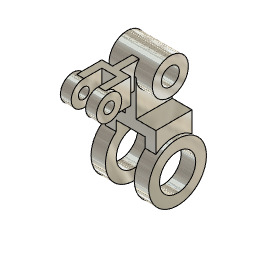
Exercise-5 v0 (Autodesk Fusion 360 design; units mm, degrees)
Autodesk Fusion 360 part; units mm, degrees
sketch "Sketch1" plane through (0, 0, 0) normal (1, 0, 0) x (0, 1, 0)
  circle A0 centre (0, 0) radius 25
  circle A1 centre (0, 0) radius 40
  circle A2 centre (0, 110) radius 12.5
  circle A3 centre (0, 110) radius 25
  circle A4 centre (-80, 110) radius 7.5
  circle A5 centre (-80, 110) radius 17.5
  dimension "d1" = 50
  dimension "d2" = 80
  dimension "d3" = 25
  dimension "d4" = 50
  dimension "d5" = 110
  dimension "d6" = 15
  dimension "d7" = 35
  dimension "d8" = 80
  constraint coincident A0.centre A1.centre
  constraint concentric A2 A3
  constraint concentric A4 A5
  measures "d1" diameter of A0
  measures "d2" diameter of A1
  measures "d3" diameter of A2
  measures "d4" diameter of A3
  measures "d5" distance of A0.centre A2.centre
  measures "d6" diameter of A4
  measures "d7" diameter of A5
  measures "d8" distance of A2.centre A4.centre
extrude "Extrude1" add sketch "Sketch1" along normal blind 20 from surface at 20 contours A1 makes body 1
extrude "Extrude2" add sketch "Sketch1" along normal blind 15 from surface at 10 separate body contours A5 makes body 2
extrude "Extrude3" add sketch "Sketch1" along normal mid plane 60 separate body contours A3 makes body 3
mirror "Mirror1" about plane through (0, 0, 0) normal (1, 0, 0) of bodies 2 1 makes body 4 at (-33.3333, 39.9503, -1.9938) makes body 5 at (-20, -62.587, 108.2576)
sketch "Sketch2" plane through (0, 0, 0) normal (0, 1, 0) x (1, 0, 0)
  line L0 (-40, -40) -> (-40, 40)
  line L1 (-20, -40) -> (-20, 40)
  line L2 (40, -40) -> (40, 40)
  line L3 (20, -40) -> (20, 40)
  line L4 (-30, -85) -> (-30, -135)
  line L5 (30, -135) -> (30, -85)
  line L6 (-20, 0) -> (-35, 0)
  line L7 (-35, 0) -> (-35, -45)
  line L8 (-35, -45) -> (-20, -45)
  line L9 (-20, -45) -> (-20, 0)
  line L10 (0, 0) -> (0, -67.4889) construction
  line L11 (35, -45) -> (20, -45)
  line L12 (35, 0) -> (35, -45)
  line L13 (20, -45) -> (20, 0)
  line L14 (20, 0) -> (35, 0)
  line L15 (-35, -45) -> (35, -45)
  line L16 (35, -45) -> (35, -60)
  line L17 (35, -60) -> (-35, -60)
  line L18 (-35, -60) -> (-35, -45)
  line L19 (-7.5, -45) -> (7.5, -45)
  line L20 (7.5, -45) -> (7.5, -110)
  line L21 (7.5, -110) -> (-7.5, -110)
  line L22 (-7.5, -110) -> (-7.5, -45)
  dimension "d19" = 15
  dimension "d20" = 45
  dimension "d21" = 15
  dimension "d22" = 15
  dimension "d23" = 65
  dimension "d24" = 27.5
  constraint horizontal L6
  constraint vertical L7
  constraint horizontal L8
  constraint vertical L9
  constraint midpoint L1 L6.start
  constraint coincident L10.start origin
  constraint vertical L10
  constraint symmetric L6.start L10 L13.end
  constraint symmetric L6.end L10 L12.start
  constraint symmetric L7.end L10 L11.start
  constraint symmetric L8.end L10 L11.end
  constraint horizontal L15
  constraint vertical L16
  constraint horizontal L17
  constraint vertical L18
  constraint collinear L12 L16
  constraint horizontal L19
  constraint vertical L20
  constraint horizontal L21
  constraint vertical L22
  constraint coincident L15 L19.start
  measures "d19" distance of L6.start L6.end
  measures "d20" distance of L6.start L8.end
  measures "d21" distance of L7.end L17.end
  measures "d22" distance of L19.start L19.end
  measures "d23" distance of L19.start L21.end
  measures "d24" distance of L16 L20
extrude "Extrude4" add sketch "Sketch2" along normal mid plane 50 separate body makes body 6
extrude "Extrude5" cut sketch "Sketch1" along normal mid plane 280 contours A0 | A2 bodies 6
ref_plane "WorkPlane1" through (17.5, -80, 110) normal (0, 0, 1) x (1, 0, 0)
sketch "Sketch3" plane through (0, 0, 110) normal (0, 0, 1) x (1, 0, 0)
  line L0 (-30, 25) -> (-30, -25)
  line L1 (30, -25) -> (30, 25)
  line L2 (-30, -25) -> (30, -25)
  line L3 (-30, 25) -> (30, 25)
  line L4 (-25, -97.5) -> (-25, -62.5)
  line L5 (-10, -97.5) -> (-10, -62.5)
  line L6 (-25, -97.5) -> (-10, -97.5)
  line L7 (-25, -62.5) -> (-10, -62.5)
  line L8 (25, -97.5) -> (25, -62.5)
  line L9 (10, -97.5) -> (10, -62.5)
  line L10 (10, -97.5) -> (25, -97.5)
  line L11 (10, -62.5) -> (25, -62.5)
  line L12 (10, -80) -> (20, -80)
  line L13 (20, -80) -> (20, -55)
  line L14 (20, -55) -> (10, -55)
  line L15 (10, -55) -> (10, -80)
  circle A0 through (10, -97.5, 0) (10, -71.25, 15.1554) (10, -71.25, -15.1554)
  line L16 (-10, -80) -> (-20, -80)
  line L17 (-20, -80) -> (-20, -55)
  line L18 (-20, -55) -> (-10, -55)
  line L19 (-10, -55) -> (-10, -80)
  line L20 (-20, -55) -> (20, -55)
  line L21 (20, -55) -> (20, -45)
  line L22 (20, -45) -> (-20, -45)
  line L23 (-20, -45) -> (-20, -55)
  line L24 (-5, -55) -> (5, -55)
  line L25 (5, -55) -> (5, 0)
  line L26 (5, 0) -> (-5, 0)
  line L27 (-5, 0) -> (-5, -55)
  dimension "d30" = 10
  dimension "d31" = 25
  dimension "d32" = 10
  dimension "d33" = 25
  dimension "d34" = 40
  dimension "d35" = 10
  dimension "d36" = 10
  dimension "d37" = 55
  dimension "d38" = 15
  constraint horizontal L12
  constraint vertical L13
  constraint horizontal L14
  constraint vertical L15
  constraint coincident L12.start L15.end
  constraint horizontal L16
  constraint vertical L17
  constraint horizontal L18
  constraint vertical L19
  constraint midpoint L5 L16.start
  constraint horizontal L20
  constraint vertical L21
  constraint horizontal L22
  constraint vertical L23
  constraint horizontal L24
  constraint vertical L25
  constraint horizontal L26
  constraint vertical L27
  constraint coincident L20 L24.start
  measures "d30" distance of L12.start L12.end
  measures "d31" distance of L12.start L14.end
  measures "d32" distance of L16.start L16.end
  measures "d33" distance of L16.start L18.end
  measures "d34" distance of L17.end L13.end
  measures "d35" distance of L17.end L22.end
  measures "d36" distance of L24.start L24.end
  measures "d37" distance of L24.start L26.end
  measures "d38" distance of L21 L25
extrude "Extrude6" add sketch "Sketch3" along normal mid plane 35 separate body contours L2 L25 L26 L27 | L2 L22 L25 L27 | L18 L20 L22 L23 L27 | L20 L22 L24 L25 L27 | L14 L20 L21 L22 L25 | L7 L17 L18 L19 L20 | L11 L13 L14 L15 L20 | L5 L7 L16 L17 L19 | L9 L11 L12 L13 L15 makes body 7
extrude "Extrude7" cut sketch "Sketch1" along normal mid plane 80 contours A2 | A4 bodies 7
combine "Combine1" operation add target body 1 tool bodies 6 7 2 5 3 4
